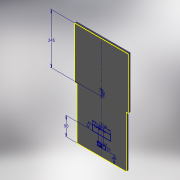
# Autodesk Inventor part: Board
Saved by Autodesk Inventor 2020 (Build 240168000, 168)
## iProperties
Created: 2019-09-17
Part Number: Board
Material: 일반
Document SubType Name: Modeling
Designer: Knowblesse
Density: 1 g/cm^3
Appearance: 기본값
Author: Knowblesse
Autodesk Inventor part; units mm, degrees
ref_plane "YZ Plane" through (0, 0, 0) normal (1, 0, 0) x (0, 1, 0)
ref_plane "XZ Plane" through (0, 0, 0) normal (0, 1, 0) x (-1, 0, 0)
ref_plane "XY Plane" through (0, 0, 0) normal (0, 0, 1) x (1, 0, 0)
sketch "스케치1" plane through (0, 0, 0) normal (0, 0, 1) x (1, 0, 0)
  line L0 (0, 0) -> (240, 0)
  line L1 (240, 0) -> (240, 250)
  line L2 (240, 250) -> (250, 250)
  line L3 (250, 250) -> (250, 500)
  line L4 (250, 500) -> (-10, 500)
  line L5 (-10, 500) -> (-10, 250)
  line L6 (-10, 250) -> (0, 250)
  line L7 (0, 250) -> (0, 0)
  dimension "d0" = 250
  dimension "d1" = 10
  dimension "d2" = 250
  dimension "d3" = 10
  dimension "d4" = 240
  constraints: 16 end point, 6 perpendicular, 2 point on line, 1 horizontal
  measures "d0" distance of L0.end L1.end
  measures "d1" distance of L1.end L2.end
  measures "d2" distance of L2.end L3.end
  measures "d3" distance of L5.end L6.end
  measures "d4" distance between parallel lines of L7 L1
extrude "돌출1" add sketch "스케치1" along normal blind 10
sketch "스케치2" plane through (0, 0, 10) normal (0, 0, 1) x (1, 0, 0)
  line L0 (0, 0) -> (240, 0) projected
  circle A0 centre (120, 45) radius 5
  point P0 (120, 0)
  dimension "d50" = 10
  dimension "d51" = 45
  constraints: 1 centre point, 1 midpoint, 1 vertical alignment
  measures "d50" diameter of A0
  measures "d51" distance of A0.centre point (120, 0)
extrude "돌출2" cut sketch "스케치2" against normal blind 10
sketch "스케치3" plane through (0, 0, 10) normal (0, 0, 1) x (1, 0, 0)
  line L0 (0, 0) -> (240, 0) projected
  line L1 (-10, 500) -> (-10, 250) projected
  line L2 (-10, 250) -> (0, 250) projected
  line L3 (0, 250) -> (0, 0) projected
  line L4 (0, 0) -> (240, 0) projected
  line L5 (240, 0) -> (240, 250) projected
  line L6 (240, 250) -> (250, 250) projected
  line L7 (250, 250) -> (250, 500) projected
  line L8 (250, 500) -> (-10, 500) projected
  line L9 (250, 500) -> (-10, 500) construction
  line L10 (120, 500) -> (120, 0) construction
  line L11 (75, 117) -> (165, 117)
  line L12 (165, 117) -> (165, 90)
  line L13 (165, 90) -> (75, 90)
  line L14 (75, 90) -> (75, 117)
  line L15 (100, 55) -> (140, 55)
  line L16 (140, 55) -> (140, 40)
  line L17 (140, 40) -> (100, 40)
  line L18 (100, 40) -> (100, 55)
  point P0 (120, 45)
  point P1 (120, 117)
  point P2 (120, 55)
  point P3 (120, 255)
  point P4 (120, 271)
  point P5 (120, 285)
  point P6 (120, 125)
  point P7 (120, 141)
  point P8 (108, 114)
  point P9 (132, 114)
  dimension "d20" = 90
  dimension "d21" = 27
  dimension "d22" = 90
  dimension "d23" = 40
  dimension "d24" = 40
  dimension "d25" = 15
  dimension "d33" = 245
  dimension "d34" = 16
  dimension "d35" = 30
  dimension "d54" = 16
  dimension "d55" = 11
  dimension "d56" = 12
  dimension "d57" = 12
  dimension "d58" = 8
  constraints: 16 end point, 4 midpoint, 4 parallel, 2 horizontal, 2 perpendicular, 1 horizontal alignment, 10 other
  measures "d20" distance of L11.start L11.end
  measures "d21" distance between parallel lines of L13 L11
  measures "d22" distance between parallel lines of L0 L13
  measures "d23" distance of L15.start L15.end
  measures "d24" distance between parallel lines of L0 L17
  measures "d25" distance between parallel lines of L15 L17
  measures "d33" distance from line of point (120, 255) L8
  measures "d34" distance of point (120, 255) point (120, 271)
  measures "d35" distance of point (120, 285) point (120, 255)
  measures "d54" distance of point (120, 141) point (120, 125)
  measures "d55" vertical distance of point (120, 125) point (108, 114)
  measures "d58" distance from line of L11 point (120, 125)
hole "구멍1" at (75, 117, 10) at (75, 90, 10) at (165, 117, 10) at (165, 90, 10) direction (0, 0, -1) diameter 3 end through all
hole "구멍2" at (100, 55, 10) at (100, 40, 10) at (140, 55, 10) at (140, 40, 10) direction (0, 0, -1) diameter 4.134 end through all thread size "M5x0.8" class "6H" standard "ISO Metric profile"
hole "구멍3" at (120, 271, 10) at (120, 255, 10) at (120, 125, 10) at (120, 141, 10) direction (0, 0, -1) diameter 3 end through all
hole "구멍4" at (120, 285, 10) at (108, 114, 10) at (132, 114, 10) direction (0, 0, -1) diameter 8 end through all
equation "\"d57\" = d56"
